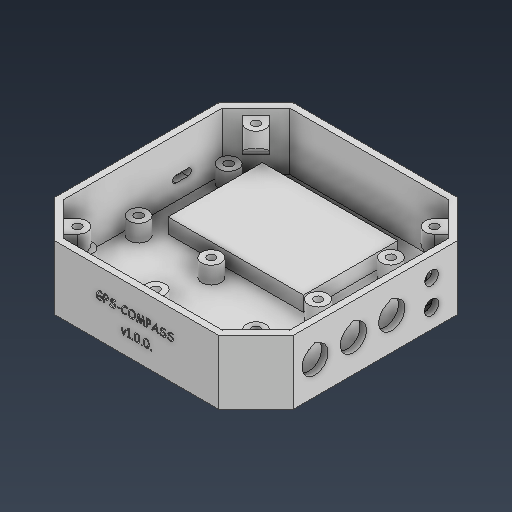
# Autodesk Inventor part: GPS-Compass_box
Saved by Autodesk Inventor 2026.2 (Build 302298000, 298)
## iProperties
Created: 2025-11-10
Part Number: GPS-Compass_box
Material: Generic
Document SubType Name: Modeling
Designer: MenMe
Density: 1 g/cm^3
Appearance: Default
Author: MenMe
Autodesk Inventor part; units mm, degrees
ref_plane "YZ Plane" through (0, 0, 0) normal (1, 0, 0) x (0, 1, 0)
ref_plane "XZ Plane" through (0, 0, 0) normal (0, 1, 0) x (-1, 0, 0)
ref_plane "XY Plane" through (0, 0, 0) normal (0, 0, 1) x (1, 0, 0)
sketch "Sketch1" plane through (0, 0, 0) normal (0, 1, 0) x (-1, 0, 0)
  line L0 (-56, 0) -> (56, 0) construction
  line L1 (0, 56) -> (0, -56) construction
  line L2 (56, 38.3223) -> (56, -38.3223)
  line L3 (56, 38.3223) -> (38.3223, 56)
  line L4 (38.3223, 56) -> (-38.3223, 56)
  line L5 (-38.3223, 56) -> (-56, 38.3223)
  line L6 (-56, 38.3223) -> (-56, -38.3223)
  line L7 (-56, -38.3223) -> (-38.3223, -56)
  line L8 (-38.3223, -56) -> (38.3223, -56)
  line L9 (38.3223, -56) -> (56, -38.3223)
  point P0 (0, 0)
  point P1 (0, 0)
  point P2 (56, 0)
  dimension "d0" = 112
  dimension "d1" = 112
  dimension "d2" = 135
  dimension "d3" = 135
  dimension "d4" = 135
  dimension "d8" = 25
  constraints: 20 end point, 7 midpoint, 2 horizontal, 2 perpendicular, 2 vertical, 1 coincident, 1 parallel
  measures "d0" distance of L0.start L0.end
  measures "d1" distance of L1.start L1.end
  measures "d2" angle of L2 L3
  measures "d3" angle of L2 L9
  measures "d4" angle of L5 L6
  measures "d8" distance of L6.end L7.end
extrude "Extrusion1" add sketch "Sketch1" along normal blind 30
sketch "Sketch2" plane through (0, 30, 0) normal (0, 1, 0) x (1, 0, 0)
  line L0 (38.3223, -56) -> (56, -38.3223) projected
  line L1 (56, -38.3223) -> (56, 38.3223) projected
  line L2 (56, 38.3223) -> (38.3223, 56) projected
  line L3 (38.3223, 56) -> (-38.3223, 56) projected
  line L4 (-38.3223, 56) -> (-56, 38.3223) projected
  line L5 (-56, 38.3223) -> (-56, -38.3223) projected
  line L6 (-56, -38.3223) -> (-38.3223, -56) projected
  line L7 (-38.3223, -56) -> (38.3223, -56) projected
  line L8 (-37.0797, 53) -> (37.0797, 53)
  line L9 (37.0797, 53) -> (53, 37.0797)
  line L10 (53, 37.0797) -> (53, -37.0797)
  line L11 (53, -37.0797) -> (37.0797, -53)
  line L12 (37.0797, -53) -> (-37.0797, -53)
  line L13 (-37.0797, -53) -> (-53, -37.0797)
  line L14 (-53, -37.0797) -> (-53, 37.0797)
  line L15 (-53, 37.0797) -> (-37.0797, 53)
  point P0 (0, 0)
  dimension "d11" = 3
  constraints: 16 end point, 7 other
  measures "d11" distance between parallel lines of L3 L8
extrude "Extrusion2" cut sketch "Sketch2" against normal blind 27 contours L8 L9 L10 L11 L12 L13 L14 L15
sketch "Sketch3" plane through (0, 3, 0) normal (0, 1, 0) x (1, 0, 0)
  circle A0 centre (-47.9582, 35.11) radius 4.5
  circle A1 centre (-47.9582, -7.09) radius 4.5
  circle A2 centre (-13.8582, -7.09) radius 4.5
  circle A3 centre (28.1418, 35.11) radius 4.5
  circle A4 centre (28.1418, 1.01) radius 4.5
  circle A5 centre (-14.0082, -33.0896) radius 4.5
  circle A6 centre (-47.8082, -33.0896) radius 4.5
  line L0 (-47.9582, -7.09) -> (-13.8582, -7.09) construction
  line L1 (-47.8082, -33.0896) -> (-14.0082, -33.0896) construction
  circle A7 centre (43.8518, 33.5) radius 4.5
  circle A8 centre (43.8518, -33.5) radius 4.5
  line L2 (37.0797, -53) -> (-37.0797, -53) projected
  line L3 (-53, -37.0797) -> (-53, 37.0797) projected
  line L4 (37.0797, 53) -> (53, 37.0797) projected
  line L5 (53, -37.0797) -> (37.0797, -53) projected
  line L6 (-10.6645, -2.1722) -> (28.1355, -2.1722)
  arc A9 (28.1355, -2.1722) -> (31.3355, 1.0278) centre (28.1355, 1.0278) ccw
  line L7 (31.3355, 35.1278) -> (31.3355, 1.0278)
  arc A10 (31.3355, 35.1278) -> (28.1355, 38.3278) centre (28.1355, 35.1278) ccw
  line L8 (6.8355, 38.3278) -> (28.1355, 38.3278)
  line L9 (6.8355, 32.6278) -> (6.8355, 38.3278)
  arc A11 (6.3355, 32.1278) -> (6.8355, 32.6278) centre (6.3355, 32.6278) ccw
  line L10 (-11.1645, 32.1278) -> (6.3355, 32.1278)
  arc A12 (-11.6645, 32.6278) -> (-11.1645, 32.1278) centre (-11.1645, 32.6278) ccw
  line L11 (-11.6645, 38.3278) -> (-11.6645, 32.6278)
  line L12 (-47.9645, 38.3278) -> (-11.6645, 38.3278)
  arc A13 (-47.9645, 38.3278) -> (-51.1645, 35.1278) centre (-47.9645, 35.1278) ccw
  line L13 (-51.1645, 35.1278) -> (-51.1645, 26.5778)
  arc A14 (-52.1645, 25.5778) -> (-51.1645, 26.5778) centre (-52.1645, 26.5778) ccw
  line L14 (-52.1645, 25.5778) -> (-52.6645, 25.5778)
  arc A15 (-52.6645, 25.5778) -> (-53.6645, 24.5778) centre (-52.6645, 24.5778) ccw
  line L15 (-53.6645, 24.5778) -> (-53.6645, 11.5778)
  arc A16 (-53.6645, 11.5778) -> (-52.6645, 10.5778) centre (-52.6645, 11.5778) ccw
  line L16 (-52.6645, 10.5778) -> (-52.1645, 10.5778)
  arc A17 (-51.1645, 9.5778) -> (-52.1645, 10.5778) centre (-52.1645, 9.5778) ccw
  line L17 (-51.1645, 9.5778) -> (-51.1645, -10.2722)
  line L18 (-51.1645, -10.2722) -> (-47.9645, -10.2722)
  arc A18 (-47.9645, -10.2722) -> (-44.7645, -7.0722) centre (-47.9645, -7.0722) ccw
  line L19 (-44.7645, -7.0722) -> (-44.7645, -6.6722)
  line L20 (-44.7645, -6.6722) -> (-17.0645, -6.6722)
  line L21 (-17.0645, -7.0722) -> (-17.0645, -6.6722)
  arc A19 (-17.0645, -7.0722) -> (-13.8645, -10.2722) centre (-13.8645, -7.0722) ccw
  line L22 (-13.8645, -10.2722) -> (-10.6645, -10.2722)
  line L23 (-10.6645, -2.1722) -> (-10.6645, -10.2722)
  line L24 (-51.1657, -10.3631) -> (-51.1657, -32.9831)
  arc A20 (-51.1657, -32.9831) -> (-47.8157, -36.3331) centre (-47.8157, -32.9831) ccw
  line L25 (-47.8157, -36.3331) -> (-14.0157, -36.3331)
  arc A21 (-14.0157, -36.3331) -> (-10.6657, -32.9831) centre (-14.0157, -32.9831) ccw
  line L26 (-10.6657, -10.3631) -> (-10.6657, -32.9831)
  line L27 (-10.6657, -10.3631) -> (-13.8657, -10.3631)
  arc A22 (-17.2157, -7.0131) -> (-13.8657, -10.3631) centre (-13.8657, -7.0131) ccw
  line L28 (-17.2157, -6.7631) -> (-17.2157, -7.0131)
  line L29 (-44.6157, -6.7631) -> (-17.2157, -6.7631)
  line L30 (-44.6157, -7.0131) -> (-44.6157, -6.7631)
  arc A23 (-47.9657, -10.3631) -> (-44.6157, -7.0131) centre (-47.9657, -7.0131) ccw
  line L31 (-51.1657, -10.3631) -> (-47.9657, -10.3631)
  arc A24 (38.8493, 37.5107) -> (36.8493, 35.5107) centre (38.8493, 35.5107) ccw
  line L32 (38.8493, 37.5107) -> (42.3493, 37.5107)
  line L33 (42.3493, 33.5107) -> (42.3493, 37.5107)
  arc A25 (42.3493, 33.5107) -> (45.3493, 33.5107) centre (43.8493, 33.5107) ccw
  line L34 (45.3493, 33.5107) -> (45.3493, 37.5107)
  line L35 (45.3493, 37.5107) -> (47.2531, 37.5107)
  line L36 (47.2531, 37.5107) -> (51.8493, 32.9145)
  line L37 (51.8493, -32.8931) -> (51.8493, 32.9145)
  line L38 (47.2531, -37.4893) -> (51.8493, -32.8931)
  line L39 (45.3493, -37.4893) -> (47.2531, -37.4893)
  line L40 (45.3493, -33.4893) -> (45.3493, -37.4893)
  arc A26 (45.3493, -33.4893) -> (42.3493, -33.4893) centre (43.8493, -33.4893) ccw
  line L41 (42.3493, -33.4893) -> (42.3493, -37.4893)
  line L42 (38.8493, -37.4893) -> (42.3493, -37.4893)
  arc A27 (36.8493, -35.4893) -> (38.8493, -37.4893) centre (38.8493, -35.4893) ccw
  line L43 (36.8493, 35.5107) -> (36.8493, -35.4893)
  point P0 (0, 0)
  point P1 (-30.9082, -33.0896)
  point P2 (-30.9082, -7.09)
  dimension "d40" = 9
  dimension "d43" = 34.1
  dimension "d58" = 76.1
  dimension "d59" = 42.2
  dimension "d60" = 34.1
  dimension "d90" = 33.8
  dimension "d105" = 26
  dimension "d128" = 9
  dimension "d135" = 67
  dimension "d144" = 34.51
  dimension "d147" = 15.71
  dimension "d264" = 9
  dimension "d265" = 9
  constraints: 80 end point, 38 point on circle, 28 centre point, 7 equal radius, 4 vertical alignment, 3 horizontal alignment, 2 horizontal, 2 midpoint
  measures "d40" diameter of A3
  measures "d43" distance of A3.centre A4.centre
  measures "d58" distance of A0.centre A3.centre
  measures "d59" distance of L0.start A0.centre
  measures "d60" distance of L0.end L0.start
  measures "d90" distance of L1.start L1.end
  measures "d105" distance of L1.end L0.end
  measures "d128" diameter of A5
  measures "d135" distance of A8.centre A7.centre
  measures "d144" vertical distance of A8.centre A4.centre
  measures "d147" horizontal distance of A7.centre A3.centre
  measures "d264" distance from line of L4 A7.centre
  measures "d265" distance from line of L5 A8.centre
extrude "Extrusion3" add sketch "Sketch3" along normal blind 8 contours A0 L13 A13 L12 | L12 A13 L13 A0 | L8 A10 L7 A3 | A3 L7 A10 L8 | L7 A9 L6 A4 | A4 L6 A9 L7 | L17 A1 | A1 L20 L19 A18 L18 L17 | A1 L29 L30 A23 L31 L18 A18 L19 L20 | A1 L31 A23 L30 L29 | L20 L21 A19 L22 A2 L27 A22 L28 L29 | A2 L23 L22 A19 L21 L20 | A2 L23 | L29 L28 A22 L27 A2 | L24 A20 L25 A6 | A6 L25 A20 L24 | L26 A21 L25 A5 | A5 L25 A21 L26 | A7 L32 L33 A25 L34 L35 | L35 L34 A25 L33 L32 A7 | L39 L40 A26 L41 L42 A8 | A8 L42 L41 A26 L40 L39
sketch "Sketch4" plane through (0, 3, 0) normal (0, 1, 0) x (1, 0, 0)
  line L0 (-41.4841, 44.4591) -> (22.0159, 44.4591)
  line L1 (22.0159, 44.4591) -> (22.0159, 0.2591)
  line L2 (22.0159, 0.2591) -> (-41.4841, 0.2591)
  line L3 (-41.4841, 0.2591) -> (-41.4841, 44.4591)
  point P0 (0, 0)
  dimension "d268" = 63.5
  dimension "d269" = 44.2
  constraints: 8 end point, 2 parallel, 1 horizontal, 1 perpendicular
  measures "d268" distance of L1.end L2.end
  measures "d269" distance of L0.end L1.end
extrude "Extrusion4" add sketch "Sketch4" along normal blind 7
sketch "Sketch5" plane through (-13.8582, 11, 7.09) normal (0, 1, 0) x (1, 0, 0)
  circle A0 centre (0, 0) radius 4.5 projected
  circle A1 centre (0, 0) radius 1.925
  circle A2 centre (-34.1, 0) radius 4.5 projected
  circle A3 centre (-34.1, 0) radius 1.925
  circle A4 centre (-34.1, 42.2) radius 4.5 projected
  circle A5 centre (-34.1, 42.2) radius 1.925
  circle A6 centre (42, 8.1) radius 4.5 projected
  circle A7 centre (42, 8.1) radius 1.925
  circle A8 centre (-33.95, -25.9996) radius 4.5 projected
  circle A9 centre (-33.95, -25.9996) radius 1.925
  circle A10 centre (-0.15, -25.9996) radius 4.5 projected
  circle A11 centre (-0.15, -25.9996) radius 1.925
  circle A12 centre (57.71, -26.41) radius 4.5 projected
  circle A13 centre (57.71, -26.41) radius 1.925
  circle A14 centre (57.71, 40.59) radius 4.5 projected
  circle A15 centre (57.71, 40.59) radius 1.925
  circle A16 centre (42, 42.2) radius 4.5 projected
  circle A17 centre (42, 42.2) radius 1.925
  point P0 (13.8582, 7.09)
  dimension "d272" = 3.85
  dimension "d273" = 3.85
  constraints: 9 centre point, 9 coincident, 7 equal radius
  measures "d272" diameter of A7
  measures "d273" diameter of A15
extrude "Extrusion5" cut sketch "Sketch5" against normal blind 5.3 contours A1 | A3 | A5 | A7 | A9 | A11 | A13 | A15 | A17
sketch "Sketch6" plane through (56, 0, 38.3223) normal (1, 0, 0) x (0, 0, -1)
  line L0 (76.6447, 0) -> (76.6447, 30) construction
  line L1 (76.6447, 15) -> (0, 15) construction
  line L2 (0, 0) -> (0, 30) construction
  arc A0 (7.0627, 20.4032) -> (12.9373, 20.4032) centre (10, 15) ccw
  line L3 (7.0627, 20.4032) -> (10, 22)
  line L4 (10, 22) -> (12.9373, 20.4032)
  arc A1 (25.0627, 20.4032) -> (30.9373, 20.4032) centre (28, 15) ccw
  line L5 (28, 22) -> (30.9373, 20.4032)
  line L6 (25.0627, 20.4032) -> (28, 22)
  arc A2 (43.0627, 20.4032) -> (48.9373, 20.4032) centre (46, 15) ccw
  line L7 (46, 22) -> (48.9373, 20.4032)
  line L8 (43.0627, 20.4032) -> (46, 22)
  circle A3 centre (64.6447, 21) radius 3.2
  circle A4 centre (64.6447, 9) radius 3.375
  point P0 (38.3223, 0)
  point P1 (52.15, 15)
  dimension "d276" = 12.3
  dimension "d277" = 7
  dimension "d280" = 18
  dimension "d285" = 10
  dimension "d288" = 6.75
  dimension "d289" = 6.4
  dimension "d290" = 12
  dimension "d291" = 6
  dimension "d292" = 6
  constraints: 14 end point, 7 point on circle, 5 centre point, 2 midpoint, 2 point on line, 2 tangent, 2 vertical alignment, 1 horizontal, 14 other
  measures "d276" diameter of A0
  measures "d277" distance of A0.centre L3.end
  measures "d280" distance of A0.centre A1.centre
  measures "d285" distance from line of L2 A0.centre
  measures "d288" diameter of A4
  measures "d289" diameter of A3
  measures "d290" distance from line of L0 A3.centre
  measures "d291" distance from line of L1 A3.centre
  measures "d292" distance from line of L1 A4.centre
extrude "Extrusion6" cut sketch "Sketch6" against normal blind 3
sketch "Sketch7" plane through (-56, 0, -38.3223) normal (-1, 0, 0) x (0, 0, 1)
  line L0 (0, 0) -> (0, 30) construction
  line L1 (76.6447, 0) -> (76.6447, 30) construction
  line L2 (17.16, 12) -> (22.84, 12) construction
  line L3 (17.16, 10.37) -> (22.84, 10.37)
  line L4 (22.84, 13.63) -> (17.16, 13.63)
  arc A0 (17.16, 13.63) -> (17.16, 10.37) centre (17.16, 12) ccw
  arc A1 (22.84, 10.37) -> (22.84, 13.63) centre (22.84, 12) ccw
  line L5 (0, 0) -> (76.6447, 0) projected
  point P0 (38.3223, 0)
  point P1 (20, 12)
  dimension "d297" = 8.94
  dimension "d298" = 3.26
  dimension "d299" = 12
  dimension "d302" = 20
  constraints: 8 end point, 4 point on circle, 4 tangent, 2 centre point, 1 horizontal, 1 midpoint, 1 parallel
  measures "d298" distance between parallel lines of L3 L4
  measures "d299" distance from line of L5 point (20, 12)
  measures "d302" distance from line of L0 point (20, 12)
extrude "Extrusion7" cut sketch "Sketch7" against normal blind 3
ref_plane "Work Plane2" through (0, 27, 0) normal (0, 1, 0) x (1, 0, 0)
sketch "Sketch8" plane through (0, 27, 0) normal (0, 1, 0) x (1, 0, 0)
  line L0 (-53, 37.0797) -> (-37.0797, 53) construction
  line L1 (-45.0398, 45.0398) -> (45.0398, -45.0398) construction
  line L2 (53, -37.0797) -> (37.0797, -53) projected
  line L3 (37.0797, 53) -> (53, 37.0797) construction
  line L4 (45.0398, 45.0398) -> (-45.0398, -45.0398) construction
  arc A0 (-45.0398, 38.6759) -> (-38.6759, 45.0398) centre (-41.8579, 41.8579) ccw
  arc A1 (38.6759, 45.0398) -> (45.0398, 38.6759) centre (41.8579, 41.8579) ccw
  arc A2 (-38.6759, -45.0398) -> (-45.0398, -38.6759) centre (-41.8579, -41.8579) ccw
  arc A3 (45.0398, -38.6759) -> (38.6759, -45.0398) centre (41.8579, -41.8579) ccw
  line L5 (-37.0797, -53) -> (-53, -37.0797) projected
  line L6 (-45.0398, 38.6759) -> (-48.2218, 41.8579)
  line L7 (-38.6759, 45.0398) -> (-41.8579, 48.2218)
  line L8 (45.0398, 38.6759) -> (48.2218, 41.8579)
  line L9 (38.6759, 45.0398) -> (41.8579, 48.2218)
  line L10 (38.6759, -45.0398) -> (41.8579, -48.2218)
  line L11 (45.0398, -38.6759) -> (48.2218, -41.8579)
  line L12 (-45.0398, -38.6759) -> (-48.2218, -41.8579)
  line L13 (-38.6759, -45.0398) -> (-41.8579, -48.2218)
  line L14 (-53, 37.0797) -> (-37.0797, 53) projected
  line L15 (37.0797, 53) -> (53, 37.0797) projected
  point P0 (0, 0)
  dimension "d303" = 9
  constraints: 20 end point, 14 point on line, 11 tangent, 8 perpendicular, 8 point on circle, 6 midpoint, 4 centre point, 3 equal radius
  measures "d303" diameter of A0
extrude "Extrusion8" add sketch "Sketch8" against normal blind 7
chamfer "Chamfer1" distance 8.99 angle 45 4 edges at (45.0398, 20, -45.0398) (45.0398, 20, 45.0398) (-45.0398, 20, 45.0398) (-45.0398, 20, -45.0398)
sketch "Sketch9" plane through (0, 27, 0) normal (0, 1, 0) x (1, 0, 0)
  arc A0 (-38.895, 38.4709) -> (-38.4709, 38.895) centre (-41.8579, 41.8579) ccw projected
  circle A1 centre (-41.8579, 41.8579) radius 1.925
  arc A2 (38.4709, 38.895) -> (38.895, 38.4709) centre (41.8579, 41.8579) ccw projected
  circle A3 centre (41.8579, 41.8579) radius 1.925
  arc A4 (-38.6759, -45.0398) -> (-45.0398, -38.6759) centre (-41.8579, -41.8579) ccw projected
  circle A5 centre (-41.8579, -41.8579) radius 1.925
  arc A6 (38.895, -38.4709) -> (38.4709, -38.895) centre (41.8579, -41.8579) ccw projected
  circle A7 centre (41.8579, -41.8579) radius 1.925
  point P0 (0, 0)
  dimension "d310" = 3.85
  constraints: 4 centre point, 4 coincident, 3 equal radius
  measures "d310" diameter of A5
extrude "Extrusion9" cut sketch "Sketch9" against normal blind 5.4
sketch "Sketch10" plane through (-38.3223, 0, 56) normal (0, 0, 1) x (1, 0, 0)
  line L0 (18.3223, 22) -> (58.3223, 22) construction
  line L1 (58.3223, 22) -> (58.3223, 6) construction
  line L2 (58.3223, 6) -> (18.3223, 6) construction
  line L3 (18.3223, 6) -> (18.3223, 22) construction
  line L4 (0, 30) -> (76.6447, 30) construction
  line L5 (38.3223, 30) -> (38.3223, 0) construction
  line L6 (76.6447, 0) -> (76.6447, 30) construction
  line L7 (76.6447, 15) -> (0, 15) construction
  line L8 (0, 0) -> (0, 30) construction
  line L9 (0, 0) -> (76.6447, 0) construction
  spline S0 degree 2 poles (22.462, 17.9114) (22.3103, 17.1528) (21.3275, 16.2459) (20.6585, 16.2459) knots 0 0 0 1 2 2 2
  spline S1 degree 2 poles (20.6585, 16.2459) (20.0482, 16.2459) (19.4413, 16.9252) (19.4413, 17.608) knots 0 0 0 1 2 2 2
  spline S2 degree 2 poles (19.4413, 17.608) (19.4413, 18.2494) (20.0482, 19.608) (20.5241, 20.0252) knots 0 0 0 1 2 2 2
  spline S3 degree 2 poles (20.5241, 20.0252) (20.8413, 20.3045) (21.193, 20.3045) knots 0 0 0 1 1 1
  spline S4 degree 2 poles (21.193, 20.3045) (21.4172, 20.3045) (21.7861, 20.1563) knots 0 0 0 1 1 1
  spline S5 degree 2 poles (21.7861, 20.1563) (22.2378, 19.977) (22.2378, 19.7632) knots 0 0 0 1 1 1
  spline S6 degree 2 poles (22.2378, 19.7632) (22.2378, 19.6597) (22.0896, 19.5011) (21.9861, 19.5011) knots 0 0 0 1 2 2 2
  spline S7 degree 2 poles (21.9861, 19.5011) (21.931, 19.5011) (21.831, 19.5632) knots 0 0 0 1 1 1
  spline S8 degree 2 poles (21.831, 19.5632) (21.4551, 19.7942) (21.193, 19.7942) knots 0 0 0 1 1 1
  spline S9 degree 2 poles (21.193, 19.7942) (21.0068, 19.7942) (20.8034, 19.6011) knots 0 0 0 1 1 1
  spline S10 degree 2 poles (20.8034, 19.6011) (20.7034, 19.5045) (20.5137, 19.2494) knots 0 0 0 1 1 1
  spline S11 degree 2 poles (20.5137, 19.2494) (19.9413, 18.4942) (19.9413, 17.608) knots 0 0 0 1 1 1
  spline S12 degree 2 poles (19.9413, 17.608) (19.9413, 17.1425) (20.0861, 16.9563) knots 0 0 0 1 1 1
  spline S13 degree 2 poles (20.0861, 16.9563) (20.2413, 16.7528) (20.6585, 16.7528) knots 0 0 0 1 1 1
  spline S14 degree 2 poles (20.6585, 16.7528) (21.0999, 16.7528) (21.4275, 17.0321) knots 0 0 0 1 1 1
  spline S15 degree 2 poles (21.4275, 17.0321) (21.7723, 17.3287) (21.9068, 17.8804) knots 0 0 0 1 1 1
  spline S16 degree 2 poles (21.9068, 17.8804) (21.2241, 17.8459) (20.7344, 17.6183) knots 0 0 0 1 1 1
  spline S17 degree 2 poles (20.7344, 17.6183) (20.6758, 17.5907) (20.6241, 17.5907) knots 0 0 0 1 1 1
  spline S18 degree 2 poles (20.6241, 17.5907) (20.5137, 17.5907) (20.4413, 17.6735) knots 0 0 0 1 1 1
  spline S19 degree 2 poles (20.4413, 17.6735) (20.3758, 17.7528) (20.3758, 17.8528) knots 0 0 0 1 1 1
  spline S20 degree 2 poles (20.3758, 17.8528) (20.3758, 17.9873) (20.5068, 18.0701) knots 0 0 0 1 1 1
  spline S21 degree 2 poles (20.5068, 18.0701) (21.0413, 18.3942) (22.3482, 18.3942) knots 0 0 0 1 1 1
  spline S22 degree 2 poles (22.3482, 18.3942) (22.4516, 18.3942) (22.5965, 18.2494) (22.5965, 18.1425) knots 0 0 0 1 2 2 2
  spline S23 degree 2 poles (22.5965, 18.1425) (22.5965, 17.9804) (22.462, 17.9114) knots 0 0 0 1 1 1
  spline S24 degree 2 poles (23.7068, 17.8701) (23.6378, 17.8701) (23.4034, 17.9011) knots 0 0 0 1 1 1
  spline S25 degree 2 poles (23.4034, 17.9011) (23.3861, 17.5287) (23.3861, 16.5942) knots 0 0 0 1 1 1
  spline S26 degree 2 poles (23.3861, 16.5942) (23.3861, 16.4942) (23.2585, 16.3597) (23.162, 16.3597) knots 0 0 0 1 2 2 2
  spline S27 degree 2 poles (23.162, 16.3597) (23.062, 16.3597) (22.9344, 16.4942) (22.9344, 16.5942) knots 0 0 0 1 2 2 2
  line L10 (22.9344, 16.5942) -> (22.9344, 17.3218)
  spline S28 degree 2 poles (22.9344, 17.3218) (22.9344, 17.6838) (22.9792, 18.3459) knots 0 0 0 1 1 1
  spline S29 degree 2 poles (22.9792, 18.3459) (23.0275, 19.0597) (23.031, 19.3701) knots 0 0 0 1 1 1
  line L11 (23.031, 19.3701) -> (23.031, 19.7114)
  spline S30 degree 2 poles (23.031, 19.7114) (23.031, 19.9563) (23.062, 20.0666) knots 0 0 0 1 1 1
  spline S31 degree 2 poles (23.062, 20.0666) (23.1206, 20.2838) (23.3034, 20.2563) knots 0 0 0 1 1 1
  spline S32 degree 2 poles (23.3034, 20.2563) (23.3827, 20.2804) (23.6758, 20.3045) (23.8896, 20.3045) knots 0 0 0 1 2 2 2
  spline S33 degree 2 poles (23.8896, 20.3045) (24.3413, 20.3045) (24.7378, 19.9942) knots 0 0 0 1 1 1
  spline S34 degree 2 poles (24.7378, 19.9942) (25.1723, 19.6528) (25.1723, 19.1735) knots 0 0 0 1 1 1
  spline S35 degree 2 poles (25.1723, 19.1735) (25.1723, 18.5597) (24.7068, 18.1976) knots 0 0 0 1 1 1
  spline S36 degree 2 poles (24.7068, 18.1976) (24.2896, 17.8701) (23.7068, 17.8701) knots 0 0 0 1 1 1
  spline S37 degree 2 poles (23.831, 19.8356) (23.7206, 19.8356) (23.5482, 19.8252) (23.4896, 19.8149) knots 0 0 0 1 2 2 2
  line L12 (23.4896, 19.8149) -> (23.4861, 19.3597)
  line L13 (23.4861, 19.3597) -> (23.4344, 18.3735)
  line L14 (23.4344, 18.3735) -> (23.7068, 18.3425)
  spline S38 degree 2 poles (23.7068, 18.3425) (24.1241, 18.3425) (24.4068, 18.5528) knots 0 0 0 1 1 1
  spline S39 degree 2 poles (24.4068, 18.5528) (24.7206, 18.7838) (24.7206, 19.1735) knots 0 0 0 1 1 1
  spline S40 degree 2 poles (24.7206, 19.1735) (24.7206, 19.4528) (24.4241, 19.6528) knots 0 0 0 1 1 1
  spline S41 degree 2 poles (24.4241, 19.6528) (24.1482, 19.8356) (23.831, 19.8356) knots 0 0 0 1 1 1
  spline S42 degree 2 poles (25.6585, 17.0321) (25.6551, 17.1356) (25.8034, 17.2666) (25.9068, 17.2666) knots 0 0 0 1 2 2 2
  spline S43 degree 2 poles (25.9068, 17.2666) (26.0275, 17.2666) (26.1206, 17.1287) knots 0 0 0 1 1 1
  spline S44 degree 2 poles (26.1206, 17.1287) (26.2482, 16.939) (26.3447, 16.8735) knots 0 0 0 1 1 1
  spline S45 degree 2 poles (26.3447, 16.8735) (26.5551, 16.7356) (26.9551, 16.7356) knots 0 0 0 1 1 1
  spline S46 degree 2 poles (26.9551, 16.7356) (27.3413, 16.7356) (27.6689, 16.9011) knots 0 0 0 1 1 1
  spline S47 degree 2 poles (27.6689, 16.9011) (28.0896, 17.1149) (28.0896, 17.4907) knots 0 0 0 1 1 1
  spline S48 degree 2 poles (28.0896, 17.4907) (28.0896, 17.8045) (27.7344, 17.9838) knots 0 0 0 1 1 1
  spline S49 degree 2 poles (27.7344, 17.9838) (27.4378, 18.139) (26.9965, 18.1528) knots 0 0 0 1 1 1
  spline S50 degree 2 poles (26.9965, 18.1528) (26.6068, 18.1666) (26.331, 18.3252) knots 0 0 0 1 1 1
  spline S51 degree 2 poles (26.331, 18.3252) (25.9792, 18.5252) (25.9792, 18.8976) knots 0 0 0 1 1 1
  spline S52 degree 2 poles (25.9792, 18.8976) (25.9792, 19.339) (26.4792, 19.7011) knots 0 0 0 1 1 1
  spline S53 degree 2 poles (26.4792, 19.7011) (26.9551, 20.0459) (27.4654, 20.0459) knots 0 0 0 1 1 1
  spline S54 degree 2 poles (27.4654, 20.0459) (27.7034, 20.0459) (28.0068, 19.9632) knots 0 0 0 1 1 1
  spline S55 degree 2 poles (28.0068, 19.9632) (28.4068, 19.8563) (28.4068, 19.6907) knots 0 0 0 1 1 1
  spline S56 degree 2 poles (28.4068, 19.6907) (28.4068, 19.4735) (28.1861, 19.4735) knots 0 0 0 1 1 1
  spline S57 degree 2 poles (28.1861, 19.4735) (28.0861, 19.4735) (27.593, 19.5804) (27.4551, 19.577) knots 0 0 0 1 2 2 2
  spline S58 degree 2 poles (27.4551, 19.577) (27.0689, 19.5735) (26.7999, 19.3873) knots 0 0 0 1 1 1
  spline S59 degree 2 poles (26.7999, 19.3873) (26.5241, 19.1976) (26.5241, 18.9252) knots 0 0 0 1 1 1
  spline S60 degree 2 poles (26.5241, 18.9252) (26.5241, 18.7218) (26.8896, 18.6356) knots 0 0 0 1 1 1
  spline S61 degree 2 poles (26.8896, 18.6356) (27.0275, 18.6045) (27.4172, 18.577) knots 0 0 0 1 1 1
  spline S62 degree 2 poles (27.4172, 18.577) (27.9827, 18.5356) (28.2999, 18.2218) knots 0 0 0 1 1 1
  spline S63 degree 2 poles (28.2999, 18.2218) (28.593, 17.9356) (28.593, 17.5218) knots 0 0 0 1 1 1
  spline S64 degree 2 poles (28.593, 17.5218) (28.593, 16.9321) (28.0482, 16.5804) knots 0 0 0 1 1 1
  spline S65 degree 2 poles (28.0482, 16.5804) (27.5758, 16.277) (26.9551, 16.277) knots 0 0 0 1 1 1
  spline S66 degree 2 poles (26.9551, 16.277) (26.4999, 16.277) (26.1275, 16.4494) knots 0 0 0 1 1 1
  spline S67 degree 2 poles (26.1275, 16.4494) (25.6654, 16.6632) (25.6585, 17.0321) knots 0 0 0 1 1 1
  spline S68 degree 2 poles (30.5172, 17.5942) (30.1827, 17.5597) (29.3206, 17.5597) knots 0 0 0 1 1 1
  spline S69 degree 2 poles (29.3206, 17.5597) (29.1137, 17.5597) (29.1137, 17.7528) knots 0 0 0 1 1 1
  spline S70 degree 2 poles (29.1137, 17.7528) (29.1137, 17.9459) (29.3206, 17.9459) knots 0 0 0 1 1 1
  spline S71 degree 2 poles (29.3206, 17.9459) (29.5172, 17.9459) (30.2999, 17.9804) (30.493, 17.9804) knots 0 0 0 1 2 2 2
  spline S72 degree 2 poles (30.493, 17.9804) (30.7137, 17.9804) (30.7137, 17.7873) knots 0 0 0 1 1 1
  spline S73 degree 2 poles (30.7137, 17.7873) (30.7137, 17.6183) (30.5172, 17.5942) knots 0 0 0 1 1 1
  spline S74 degree 2 poles (33.6792, 19.1907) (33.5206, 19.1907) (33.4413, 19.377) knots 0 0 0 1 1 1
  spline S75 degree 2 poles (33.4413, 19.377) (33.3723, 19.5356) (33.3137, 19.5701) knots 0 0 0 1 1 1
  spline S76 degree 2 poles (33.3137, 19.5701) (33.262, 19.5976) (33.0551, 19.5976) knots 0 0 0 1 1 1
  spline S77 degree 2 poles (33.0551, 19.5976) (32.6965, 19.5976) (32.2585, 19.0494) knots 0 0 0 1 1 1
  spline S78 degree 2 poles (32.2585, 19.0494) (31.6654, 18.3114) (31.6654, 17.6528) knots 0 0 0 1 1 1
  spline S79 degree 2 poles (31.6654, 17.6528) (31.6654, 17.3321) (31.8723, 17.1045) knots 0 0 0 1 1 1
  spline S80 degree 2 poles (31.8723, 17.1045) (32.0827, 16.8666) (32.3792, 16.8666) knots 0 0 0 1 1 1
  spline S81 degree 2 poles (32.3792, 16.8666) (32.6344, 16.8666) (32.8896, 16.9976) knots 0 0 0 1 1 1
  spline S82 degree 2 poles (32.8896, 16.9976) (33.0344, 17.0735) (33.331, 17.2907) knots 0 0 0 1 1 1
  spline S83 degree 2 poles (33.331, 17.2907) (33.4723, 17.3942) (33.5447, 17.3942) knots 0 0 0 1 1 1
  spline S84 degree 2 poles (33.5447, 17.3942) (33.6482, 17.3942) (33.793, 17.2321) (33.793, 17.1356) knots 0 0 0 1 2 2 2
  spline S85 degree 2 poles (33.793, 17.1356) (33.793, 17.0218) (33.6999, 16.939) knots 0 0 0 1 1 1
  spline S86 degree 2 poles (33.6999, 16.939) (33.0447, 16.3597) (32.3792, 16.3597) knots 0 0 0 1 1 1
  spline S87 degree 2 poles (32.3792, 16.3597) (31.8654, 16.3597) (31.5137, 16.7528) knots 0 0 0 1 1 1
  spline S88 degree 2 poles (31.5137, 16.7528) (31.1723, 17.1321) (31.1723, 17.6528) knots 0 0 0 1 1 1
  spline S89 degree 2 poles (31.1723, 17.6528) (31.1723, 18.4907) (31.8758, 19.3701) knots 0 0 0 1 1 1
  spline S90 degree 2 poles (31.8758, 19.3701) (32.462, 20.1045) (33.0551, 20.1045) knots 0 0 0 1 1 1
  spline S91 degree 2 poles (33.0551, 20.1045) (33.1758, 20.1045) (33.3689, 20.0838) (33.4447, 20.0563) knots 0 0 0 1 2 2 2
  spline S92 degree 2 poles (33.4447, 20.0563) (33.531, 20.1838) (33.6689, 20.1838) knots 0 0 0 1 1 1
  spline S93 degree 2 poles (33.6689, 20.1838) (33.8413, 20.1838) (33.8861, 19.9597) knots 0 0 0 1 1 1
  spline S94 degree 2 poles (33.8861, 19.9597) (33.9241, 19.7563) (33.9241, 19.4666) knots 0 0 0 1 1 1
  spline S95 degree 2 poles (33.9241, 19.4666) (33.9241, 19.3632) (33.8689, 19.2873) knots 0 0 0 1 1 1
  spline S96 degree 2 poles (33.8689, 19.2873) (33.8034, 19.1907) (33.6792, 19.1907) knots 0 0 0 1 1 1
  spline S97 degree 2 poles (35.9827, 16.2666) (35.2861, 16.2666) (34.7999, 16.6838) knots 0 0 0 1 1 1
  spline S98 degree 2 poles (34.7999, 16.6838) (34.2861, 17.1287) (34.2861, 17.8321) knots 0 0 0 1 1 1
  spline S99 degree 2 poles (34.2861, 17.8321) (34.2861, 18.6907) (34.793, 19.3907) knots 0 0 0 1 1 1
  spline S100 degree 2 poles (34.793, 19.3907) (35.3585, 20.1666) (36.2068, 20.1666) knots 0 0 0 1 1 1
  spline S101 degree 2 poles (36.2068, 20.1666) (37.0172, 20.1666) (37.4137, 19.8011) knots 0 0 0 1 1 1
  spline S102 degree 2 poles (37.4137, 19.8011) (37.8275, 19.4183) (37.8275, 18.5976) knots 0 0 0 1 1 1
  spline S103 degree 2 poles (37.8275, 18.5976) (37.8275, 17.7425) (37.362, 17.0528) knots 0 0 0 1 1 1
  spline S104 degree 2 poles (37.362, 17.0528) (36.8275, 16.2666) (35.9827, 16.2666) knots 0 0 0 1 1 1
  spline S105 degree 2 poles (36.2068, 19.6597) (35.5999, 19.6597) (35.1792, 19.0563) knots 0 0 0 1 1 1
  spline S106 degree 2 poles (35.1792, 19.0563) (34.7896, 18.5011) (34.7896, 17.8321) knots 0 0 0 1 1 1
  spline S107 degree 2 poles (34.7896, 17.8321) (34.7896, 17.3563) (35.1447, 17.0563) knots 0 0 0 1 1 1
  spline S108 degree 2 poles (35.1447, 17.0563) (35.4827, 16.7735) (35.9827, 16.7735) knots 0 0 0 1 1 1
  spline S109 degree 2 poles (35.9827, 16.7735) (36.5827, 16.7735) (36.9758, 17.3804) knots 0 0 0 1 1 1
  spline S110 degree 2 poles (36.9758, 17.3804) (37.3241, 17.9218) (37.3241, 18.5976) knots 0 0 0 1 1 1
  spline S111 degree 2 poles (37.3241, 18.5976) (37.3241, 19.1907) (37.0585, 19.4287) knots 0 0 0 1 1 1
  spline S112 degree 2 poles (37.0585, 19.4287) (36.8068, 19.6597) (36.2068, 19.6597) knots 0 0 0 1 1 1
  spline S113 degree 2 poles (42.062, 16.2114) (41.9275, 16.2114) (41.8413, 16.3494) knots 0 0 0 1 1 1
  spline S114 degree 2 poles (41.8413, 16.3494) (41.7689, 16.4701) (41.7103, 16.7459) knots 0 0 0 1 1 1
  line L15 (41.7103, 16.7459) -> (41.6206, 17.1735)
  spline S115 degree 2 poles (41.6206, 17.1735) (41.5172, 17.5701) (41.2999, 18.9183) knots 0 0 0 1 1 1
  line L16 (41.2999, 18.9183) -> (40.8034, 17.4287)
  line L17 (40.8034, 17.4287) -> (40.6585, 16.9563)
  spline S116 degree 2 poles (40.6585, 16.9563) (40.5689, 16.677) (40.4723, 16.5011) knots 0 0 0 1 1 1
  spline S117 degree 2 poles (40.4723, 16.5011) (40.3689, 16.3114) (40.193, 16.3114) knots 0 0 0 1 1 1
  spline S118 degree 2 poles (40.193, 16.3114) (40.0447, 16.3114) (39.962, 16.4701) knots 0 0 0 1 1 1
  spline S119 degree 2 poles (39.962, 16.4701) (39.9068, 16.5735) (39.862, 16.7356) knots 0 0 0 1 1 1
  line L18 (39.862, 16.7356) -> (39.7896, 17.008)
  spline S120 degree 2 poles (39.7896, 17.008) (39.5413, 17.8838) (39.3516, 18.8804) knots 0 0 0 1 1 1
  line L19 (39.3516, 18.8804) -> (39.262, 18.4356)
  line L20 (39.262, 18.4356) -> (38.9413, 17.1287)
  spline S121 degree 2 poles (38.9413, 17.1287) (38.9241, 16.9011) (38.8206, 16.4494) knots 0 0 0 1 1 1
  spline S122 degree 2 poles (38.8206, 16.4494) (38.7447, 16.2563) (38.5758, 16.2563) knots 0 0 0 1 1 1
  spline S123 degree 2 poles (38.5758, 16.2563) (38.4551, 16.2563) (38.3827, 16.3425) knots 0 0 0 1 1 1
  spline S124 degree 2 poles (38.3827, 16.3425) (38.3206, 16.4183) (38.3206, 16.5252) knots 0 0 0 1 1 1
  spline S125 degree 2 poles (38.3206, 16.5252) (38.3206, 16.939) (38.4896, 17.5425) knots 0 0 0 1 1 1
  line L21 (38.4896, 17.5425) -> (38.762, 18.539)
  line L22 (38.762, 18.539) -> (38.9068, 19.3183)
  spline S126 degree 2 poles (38.9068, 19.3183) (39.0137, 19.8666) (39.1344, 20.0321) knots 0 0 0 1 1 1
  spline S127 degree 2 poles (39.1344, 20.0321) (39.2344, 20.177) (39.3792, 20.177) knots 0 0 0 1 1 1
  spline S128 degree 2 poles (39.3792, 20.177) (39.5413, 20.177) (39.6206, 19.9942) knots 0 0 0 1 1 1
  spline S129 degree 2 poles (39.6206, 19.9942) (39.7172, 19.7735) (39.8275, 19.0942) knots 0 0 0 1 1 1
  spline S130 degree 2 poles (39.8275, 19.0942) (39.9585, 18.2804) (40.2378, 17.3321) knots 0 0 0 1 1 1
  spline S131 degree 2 poles (40.2378, 17.3321) (40.6034, 18.2873) (40.8689, 19.3183) knots 0 0 0 1 1 1
  line L23 (40.8689, 19.3183) -> (40.9447, 19.6804)
  spline S132 degree 2 poles (40.9447, 19.6804) (40.9896, 19.8976) (41.062, 20.0321) knots 0 0 0 1 1 1
  spline S133 degree 2 poles (41.062, 20.0321) (41.1585, 20.2114) (41.3241, 20.2114) knots 0 0 0 1 1 1
  spline S134 degree 2 poles (41.3241, 20.2114) (41.5378, 20.2114) (41.6482, 19.8045) knots 0 0 0 1 1 1
  spline S135 degree 2 poles (41.6482, 19.8045) (41.6896, 19.6632) (41.7447, 19.2183) knots 0 0 0 1 1 1
  spline S136 degree 2 poles (41.7447, 19.2183) (41.893, 18.1011) (42.1103, 17.308) knots 0 0 0 1 1 1
  line L24 (42.1103, 17.308) -> (42.231, 16.8838)
  spline S137 degree 2 poles (42.231, 16.8838) (42.3241, 16.5425) (42.3241, 16.4632) knots 0 0 0 1 1 1
  spline S138 degree 2 poles (42.3241, 16.4632) (42.3241, 16.3563) (42.162, 16.2114) (42.062, 16.2114) knots 0 0 0 1 2 2 2
  spline S139 degree 2 poles (43.5378, 17.8701) (43.4689, 17.8701) (43.2344, 17.9011) knots 0 0 0 1 1 1
  spline S140 degree 2 poles (43.2344, 17.9011) (43.2172, 17.5287) (43.2172, 16.5942) knots 0 0 0 1 1 1
  spline S141 degree 2 poles (43.2172, 16.5942) (43.2172, 16.4942) (43.0896, 16.3597) (42.993, 16.3597) knots 0 0 0 1 2 2 2
  spline S142 degree 2 poles (42.993, 16.3597) (42.893, 16.3597) (42.7654, 16.4942) (42.7654, 16.5942) knots 0 0 0 1 2 2 2
  line L25 (42.7654, 16.5942) -> (42.7654, 17.3218)
  spline S143 degree 2 poles (42.7654, 17.3218) (42.7654, 17.6838) (42.8103, 18.3459) knots 0 0 0 1 1 1
  spline S144 degree 2 poles (42.8103, 18.3459) (42.8585, 19.0597) (42.862, 19.3701) knots 0 0 0 1 1 1
  line L26 (42.862, 19.3701) -> (42.862, 19.7114)
  spline S145 degree 2 poles (42.862, 19.7114) (42.862, 19.9563) (42.893, 20.0666) knots 0 0 0 1 1 1
  spline S146 degree 2 poles (42.893, 20.0666) (42.9516, 20.2838) (43.1344, 20.2563) knots 0 0 0 1 1 1
  spline S147 degree 2 poles (43.1344, 20.2563) (43.2137, 20.2804) (43.5068, 20.3045) (43.7206, 20.3045) knots 0 0 0 1 2 2 2
  spline S148 degree 2 poles (43.7206, 20.3045) (44.1723, 20.3045) (44.5689, 19.9942) knots 0 0 0 1 1 1
  spline S149 degree 2 poles (44.5689, 19.9942) (45.0034, 19.6528) (45.0034, 19.1735) knots 0 0 0 1 1 1
  spline S150 degree 2 poles (45.0034, 19.1735) (45.0034, 18.5597) (44.5378, 18.1976) knots 0 0 0 1 1 1
  spline S151 degree 2 poles (44.5378, 18.1976) (44.1206, 17.8701) (43.5378, 17.8701) knots 0 0 0 1 1 1
  spline S152 degree 2 poles (43.662, 19.8356) (43.5516, 19.8356) (43.3792, 19.8252) (43.3206, 19.8149) knots 0 0 0 1 2 2 2
  line L27 (43.3206, 19.8149) -> (43.3172, 19.3597)
  line L28 (43.3172, 19.3597) -> (43.2654, 18.3735)
  line L29 (43.2654, 18.3735) -> (43.5378, 18.3425)
  spline S153 degree 2 poles (43.5378, 18.3425) (43.9551, 18.3425) (44.2378, 18.5528) knots 0 0 0 1 1 1
  spline S154 degree 2 poles (44.2378, 18.5528) (44.5516, 18.7838) (44.5516, 19.1735) knots 0 0 0 1 1 1
  spline S155 degree 2 poles (44.5516, 19.1735) (44.5516, 19.4528) (44.2551, 19.6528) knots 0 0 0 1 1 1
  spline S156 degree 2 poles (44.2551, 19.6528) (43.9792, 19.8356) (43.662, 19.8356) knots 0 0 0 1 1 1
  spline S157 degree 2 poles (48.2482, 16.3425) (48.0206, 16.3425) (47.8516, 16.9252) knots 0 0 0 1 1 1
  spline S158 degree 2 poles (47.8516, 16.9252) (47.7861, 17.1494) (47.6896, 17.7045) knots 0 0 0 1 1 1
  spline S159 degree 2 poles (47.6896, 17.7045) (47.4378, 17.6701) (47.031, 17.5804) knots 0 0 0 1 1 1
  line L30 (47.031, 17.5804) -> (46.3758, 17.4459)
  spline S160 degree 2 poles (46.3758, 17.4459) (46.2516, 17.1218) (45.9482, 16.4976) knots 0 0 0 1 1 1
  spline S161 degree 2 poles (45.9482, 16.4976) (45.8689, 16.3597) (45.7344, 16.3597) knots 0 0 0 1 1 1
  spline S162 degree 2 poles (45.7344, 16.3597) (45.6344, 16.3597) (45.4792, 16.5045) (45.4792, 16.608) knots 0 0 0 1 2 2 2
  spline S163 degree 2 poles (45.4792, 16.608) (45.4792, 16.7287) (45.8516, 17.5114) knots 0 0 0 1 1 1
  spline S164 degree 2 poles (45.8516, 17.5114) (45.8103, 17.577) (45.8103, 17.6597) knots 0 0 0 1 1 1
  spline S165 degree 2 poles (45.8103, 17.6597) (45.8103, 17.8597) (46.0516, 17.9183) knots 0 0 0 1 1 1
  spline S166 degree 2 poles (46.0516, 17.9183) (46.3344, 18.4459) (46.7654, 19.1356) knots 0 0 0 1 1 1
  spline S167 degree 2 poles (46.7654, 19.1356) (47.3516, 20.0735) (47.4965, 20.0735) knots 0 0 0 1 1 1
  spline S168 degree 2 poles (47.4965, 20.0735) (47.6896, 20.0735) (47.762, 19.8011) knots 0 0 0 1 1 1
  line L31 (47.762, 19.8011) -> (47.9172, 18.9701)
  line L32 (47.9172, 18.9701) -> (48.2861, 17.2494)
  line L33 (48.2861, 17.2494) -> (48.4275, 16.8597)
  spline S169 degree 2 poles (48.4275, 16.8597) (48.4999, 16.6597) (48.4999, 16.5907) knots 0 0 0 1 1 1
  spline S170 degree 2 poles (48.4999, 16.5907) (48.4999, 16.4873) (48.3482, 16.3425) (48.2482, 16.3425) knots 0 0 0 1 2 2 2
  line L34 (47.3758, 19.1701) -> (46.6689, 18.0287)
  spline S171 degree 2 poles (46.6689, 18.0287) (46.9689, 18.1045) (47.5758, 18.2149) knots 0 0 0 1 1 1
  line L35 (47.5758, 18.2149) -> (47.3758, 19.1701)
  spline S172 degree 2 poles (49.193, 17.0321) (49.1896, 17.1356) (49.3378, 17.2666) (49.4413, 17.2666) knots 0 0 0 1 2 2 2
  spline S173 degree 2 poles (49.4413, 17.2666) (49.562, 17.2666) (49.6551, 17.1287) knots 0 0 0 1 1 1
  spline S174 degree 2 poles (49.6551, 17.1287) (49.7827, 16.939) (49.8792, 16.8735) knots 0 0 0 1 1 1
  spline S175 degree 2 poles (49.8792, 16.8735) (50.0896, 16.7356) (50.4896, 16.7356) knots 0 0 0 1 1 1
  spline S176 degree 2 poles (50.4896, 16.7356) (50.8758, 16.7356) (51.2034, 16.9011) knots 0 0 0 1 1 1
  spline S177 degree 2 poles (51.2034, 16.9011) (51.6241, 17.1149) (51.6241, 17.4907) knots 0 0 0 1 1 1
  spline S178 degree 2 poles (51.6241, 17.4907) (51.6241, 17.8045) (51.2689, 17.9838) knots 0 0 0 1 1 1
  spline S179 degree 2 poles (51.2689, 17.9838) (50.9723, 18.139) (50.531, 18.1528) knots 0 0 0 1 1 1
  spline S180 degree 2 poles (50.531, 18.1528) (50.1413, 18.1666) (49.8654, 18.3252) knots 0 0 0 1 1 1
  spline S181 degree 2 poles (49.8654, 18.3252) (49.5137, 18.5252) (49.5137, 18.8976) knots 0 0 0 1 1 1
  spline S182 degree 2 poles (49.5137, 18.8976) (49.5137, 19.339) (50.0137, 19.7011) knots 0 0 0 1 1 1
  spline S183 degree 2 poles (50.0137, 19.7011) (50.4896, 20.0459) (50.9999, 20.0459) knots 0 0 0 1 1 1
  spline S184 degree 2 poles (50.9999, 20.0459) (51.2378, 20.0459) (51.5413, 19.9632) knots 0 0 0 1 1 1
  spline S185 degree 2 poles (51.5413, 19.9632) (51.9413, 19.8563) (51.9413, 19.6907) knots 0 0 0 1 1 1
  spline S186 degree 2 poles (51.9413, 19.6907) (51.9413, 19.4735) (51.7206, 19.4735) knots 0 0 0 1 1 1
  spline S187 degree 2 poles (51.7206, 19.4735) (51.6206, 19.4735) (51.1275, 19.5804) (50.9896, 19.577) knots 0 0 0 1 2 2 2
  spline S188 degree 2 poles (50.9896, 19.577) (50.6034, 19.5735) (50.3344, 19.3873) knots 0 0 0 1 1 1
  spline S189 degree 2 poles (50.3344, 19.3873) (50.0585, 19.1976) (50.0585, 18.9252) knots 0 0 0 1 1 1
  spline S190 degree 2 poles (50.0585, 18.9252) (50.0585, 18.7218) (50.4241, 18.6356) knots 0 0 0 1 1 1
  spline S191 degree 2 poles (50.4241, 18.6356) (50.562, 18.6045) (50.9516, 18.577) knots 0 0 0 1 1 1
  spline S192 degree 2 poles (50.9516, 18.577) (51.5172, 18.5356) (51.8344, 18.2218) knots 0 0 0 1 1 1
  spline S193 degree 2 poles (51.8344, 18.2218) (52.1275, 17.9356) (52.1275, 17.5218) knots 0 0 0 1 1 1
  spline S194 degree 2 poles (52.1275, 17.5218) (52.1275, 16.9321) (51.5827, 16.5804) knots 0 0 0 1 1 1
  spline S195 degree 2 poles (51.5827, 16.5804) (51.1103, 16.277) (50.4896, 16.277) knots 0 0 0 1 1 1
  spline S196 degree 2 poles (50.4896, 16.277) (50.0344, 16.277) (49.662, 16.4494) knots 0 0 0 1 1 1
  spline S197 degree 2 poles (49.662, 16.4494) (49.1999, 16.6632) (49.193, 17.0321) knots 0 0 0 1 1 1
  spline S198 degree 2 poles (52.7068, 17.0321) (52.7034, 17.1356) (52.8516, 17.2666) (52.9551, 17.2666) knots 0 0 0 1 2 2 2
  spline S199 degree 2 poles (52.9551, 17.2666) (53.0758, 17.2666) (53.1689, 17.1287) knots 0 0 0 1 1 1
  spline S200 degree 2 poles (53.1689, 17.1287) (53.2965, 16.939) (53.393, 16.8735) knots 0 0 0 1 1 1
  spline S201 degree 2 poles (53.393, 16.8735) (53.6034, 16.7356) (54.0034, 16.7356) knots 0 0 0 1 1 1
  spline S202 degree 2 poles (54.0034, 16.7356) (54.3896, 16.7356) (54.7172, 16.9011) knots 0 0 0 1 1 1
  spline S203 degree 2 poles (54.7172, 16.9011) (55.1378, 17.1149) (55.1378, 17.4907) knots 0 0 0 1 1 1
  spline S204 degree 2 poles (55.1378, 17.4907) (55.1378, 17.8045) (54.7827, 17.9838) knots 0 0 0 1 1 1
  spline S205 degree 2 poles (54.7827, 17.9838) (54.4861, 18.139) (54.0447, 18.1528) knots 0 0 0 1 1 1
  spline S206 degree 2 poles (54.0447, 18.1528) (53.6551, 18.1666) (53.3792, 18.3252) knots 0 0 0 1 1 1
  spline S207 degree 2 poles (53.3792, 18.3252) (53.0275, 18.5252) (53.0275, 18.8976) knots 0 0 0 1 1 1
  spline S208 degree 2 poles (53.0275, 18.8976) (53.0275, 19.339) (53.5275, 19.7011) knots 0 0 0 1 1 1
  spline S209 degree 2 poles (53.5275, 19.7011) (54.0034, 20.0459) (54.5137, 20.0459) knots 0 0 0 1 1 1
  spline S210 degree 2 poles (54.5137, 20.0459) (54.7516, 20.0459) (55.0551, 19.9632) knots 0 0 0 1 1 1
  spline S211 degree 2 poles (55.0551, 19.9632) (55.4551, 19.8563) (55.4551, 19.6907) knots 0 0 0 1 1 1
  spline S212 degree 2 poles (55.4551, 19.6907) (55.4551, 19.4735) (55.2344, 19.4735) knots 0 0 0 1 1 1
  spline S213 degree 2 poles (55.2344, 19.4735) (55.1344, 19.4735) (54.6413, 19.5804) (54.5034, 19.577) knots 0 0 0 1 2 2 2
  spline S214 degree 2 poles (54.5034, 19.577) (54.1172, 19.5735) (53.8482, 19.3873) knots 0 0 0 1 1 1
  spline S215 degree 2 poles (53.8482, 19.3873) (53.5723, 19.1976) (53.5723, 18.9252) knots 0 0 0 1 1 1
  spline S216 degree 2 poles (53.5723, 18.9252) (53.5723, 18.7218) (53.9378, 18.6356) knots 0 0 0 1 1 1
  spline S217 degree 2 poles (53.9378, 18.6356) (54.0758, 18.6045) (54.4654, 18.577) knots 0 0 0 1 1 1
  spline S218 degree 2 poles (54.4654, 18.577) (55.031, 18.5356) (55.3482, 18.2218) knots 0 0 0 1 1 1
  spline S219 degree 2 poles (55.3482, 18.2218) (55.6413, 17.9356) (55.6413, 17.5218) knots 0 0 0 1 1 1
  spline S220 degree 2 poles (55.6413, 17.5218) (55.6413, 16.9321) (55.0965, 16.5804) knots 0 0 0 1 1 1
  spline S221 degree 2 poles (55.0965, 16.5804) (54.6241, 16.277) (54.0034, 16.277) knots 0 0 0 1 1 1
  spline S222 degree 2 poles (54.0034, 16.277) (53.5482, 16.277) (53.1758, 16.4494) knots 0 0 0 1 1 1
  spline S223 degree 2 poles (53.1758, 16.4494) (52.7137, 16.6632) (52.7068, 17.0321) knots 0 0 0 1 1 1
  spline S224 degree 2 poles (32.4482, 8.0541) (32.4413, 7.8265) (32.2241, 7.8265) knots 0 0 0 1 1 1
  spline S225 degree 2 poles (32.2241, 7.8265) (32.0413, 7.8265) (31.962, 8.0403) knots 0 0 0 1 1 1
  line L36 (31.962, 8.0403) -> (31.5827, 9.0437)
  line L37 (31.5827, 9.0437) -> (31.1413, 10.1782)
  spline S226 degree 2 poles (31.1413, 10.1782) (31.1172, 10.2437) (31.1172, 10.292) knots 0 0 0 1 1 1
  spline S227 degree 2 poles (31.1172, 10.292) (31.1172, 10.3955) (31.2723, 10.5368) (31.3723, 10.5368) knots 0 0 0 1 2 2 2
  spline S228 degree 2 poles (31.3723, 10.5368) (31.5206, 10.5368) (31.5861, 10.3886) knots 0 0 0 1 1 1
  line L38 (31.5861, 10.3886) -> (32.2137, 8.6575)
  spline S229 degree 2 poles (32.2137, 8.6575) (32.3999, 9.0541) (32.6792, 9.8058) knots 0 0 0 1 1 1
  spline S230 degree 2 poles (32.6792, 9.8058) (32.7482, 10.0024) (32.8896, 10.3644) knots 0 0 0 1 1 1
  spline S231 degree 2 poles (32.8896, 10.3644) (32.9654, 10.523) (33.1068, 10.523) knots 0 0 0 1 1 1
  spline S232 degree 2 poles (33.1068, 10.523) (33.2103, 10.523) (33.362, 10.3782) (33.362, 10.2817) knots 0 0 0 1 2 2 2
  spline S233 degree 2 poles (33.362, 10.2817) (33.362, 10.1851) (32.9551, 9.223) knots 0 0 0 1 1 1
  line L39 (32.9551, 9.223) -> (32.4482, 8.0541)
  line L40 (35.1689, 7.923) -> (34.6792, 7.923)
  line L41 (34.6792, 7.923) -> (34.1896, 7.9265)
  spline S234 degree 2 poles (34.1896, 7.9265) (34.0172, 7.9265) (33.9482, 7.9472) knots 0 0 0 1 1 1
  spline S235 degree 2 poles (33.9482, 7.9472) (33.8206, 7.992) (33.8206, 8.1368) knots 0 0 0 1 1 1
  spline S236 degree 2 poles (33.8206, 8.1368) (33.8206, 8.3851) (34.2068, 8.3851) knots 0 0 0 1 1 1
  line L42 (34.2068, 8.3851) -> (34.3275, 8.3817)
  line L43 (34.3275, 8.3817) -> (34.4275, 8.3782)
  spline S237 degree 2 poles (34.4275, 8.3782) (34.4275, 8.4955) (34.3861, 8.961) (34.3861, 9.0782) knots 0 0 0 1 2 2 2
  spline S238 degree 2 poles (34.3861, 9.0782) (34.3861, 9.392) (34.4413, 10.0334) knots 0 0 0 1 1 1
  spline S239 degree 2 poles (34.4413, 10.0334) (34.4965, 10.661) (34.493, 10.9886) knots 0 0 0 1 1 1
  spline S240 degree 2 poles (34.493, 10.9886) (34.162, 10.7299) (34.0723, 10.7299) knots 0 0 0 1 1 1
  spline S241 degree 2 poles (34.0723, 10.7299) (33.9723, 10.7299) (33.8275, 10.8782) (33.8275, 10.9748) knots 0 0 0 1 2 2 2
  spline S242 degree 2 poles (33.8275, 10.9748) (33.8275, 11.092) (34.0413, 11.2575) knots 0 0 0 1 1 1
  spline S243 degree 2 poles (34.0413, 11.2575) (34.1723, 11.3541) (34.4172, 11.561) knots 0 0 0 1 1 1
  spline S244 degree 2 poles (34.4172, 11.561) (34.6378, 11.7817) (34.8344, 11.7817) knots 0 0 0 1 1 1
  spline S245 degree 2 poles (34.8344, 11.7817) (34.9999, 11.7817) (34.9999, 11.592) knots 0 0 0 1 1 1
  spline S246 degree 2 poles (34.9999, 11.592) (34.9999, 11.5334) (34.9689, 11.3093) (34.9689, 11.2506) knots 0 0 0 1 2 2 2
  spline S247 degree 2 poles (34.9689, 11.2506) (34.9689, 11.1713) (34.9861, 10.8403) (34.9861, 10.7575) knots 0 0 0 1 2 2 2
  spline S248 degree 2 poles (34.9861, 10.7575) (34.9861, 10.4748) (34.8689, 9.3575) (34.8689, 9.0782) knots 0 0 0 1 2 2 2
  spline S249 degree 2 poles (34.8689, 9.0782) (34.8689, 8.9334) (34.9068, 8.523) (34.9103, 8.392) knots 0 0 0 1 2 2 2
  line L44 (34.9103, 8.392) -> (35.1689, 8.3955)
  spline S250 degree 2 poles (35.1689, 8.3955) (35.2758, 8.3955) (35.4103, 8.261) (35.4103, 8.161) knots 0 0 0 1 2 2 2
  spline S251 degree 2 poles (35.4103, 8.161) (35.4103, 8.0575) (35.2758, 7.923) (35.1689, 7.923) knots 0 0 0 1 2 2 2
  spline S252 degree 2 poles (36.3689, 7.6955) (36.2413, 7.6955) (36.062, 7.8748) (36.062, 8.0024) knots 0 0 0 1 2 2 2
  spline S253 degree 2 poles (36.062, 8.0024) (36.062, 8.1299) (36.2413, 8.3093) (36.3689, 8.3093) knots 0 0 0 1 2 2 2
  spline S254 degree 2 poles (36.3689, 8.3093) (36.4965, 8.3093) (36.6758, 8.1299) (36.6758, 8.0024) knots 0 0 0 1 2 2 2
  spline S255 degree 2 poles (36.6758, 8.0024) (36.6758, 7.8748) (36.4965, 7.6955) (36.3689, 7.6955) knots 0 0 0 1 2 2 2
  spline S256 degree 2 poles (38.4827, 7.8299) (37.731, 7.8299) (37.3861, 8.5162) knots 0 0 0 1 1 1
  spline S257 degree 2 poles (37.3861, 8.5162) (37.1241, 9.0472) (37.1241, 9.8955) knots 0 0 0 1 1 1
  spline S258 degree 2 poles (37.1241, 9.8955) (37.1241, 10.6127) (37.4654, 11.1472) knots 0 0 0 1 1 1
  spline S259 degree 2 poles (37.4654, 11.1472) (37.8689, 11.7713) (38.5585, 11.7713) knots 0 0 0 1 1 1
  spline S260 degree 2 poles (38.5585, 11.7713) (39.2103, 11.7713) (39.5723, 11.2162) knots 0 0 0 1 1 1
  spline S261 degree 2 poles (39.5723, 11.2162) (39.8861, 10.7368) (39.8861, 10.0472) knots 0 0 0 1 1 1
  spline S262 degree 2 poles (39.8861, 10.0472) (39.8861, 8.9403) (39.1861, 7.8299) (38.4827, 7.8299) knots 0 0 0 1 2 2 2
  spline S263 degree 2 poles (38.5585, 11.2955) (38.0965, 11.2955) (37.8275, 10.8265) knots 0 0 0 1 1 1
  spline S264 degree 2 poles (37.8275, 10.8265) (37.6034, 10.4368) (37.6034, 9.9368) knots 0 0 0 1 1 1
  spline S265 degree 2 poles (37.6034, 9.9368) (37.6034, 9.123) (38.0447, 8.3058) (38.4827, 8.3058) knots 0 0 0 1 2 2 2
  spline S266 degree 2 poles (38.4827, 8.3058) (39.0068, 8.3058) (39.2344, 8.9058) knots 0 0 0 1 1 1
  spline S267 degree 2 poles (39.2344, 8.9058) (39.393, 9.3196) (39.393, 9.9575) knots 0 0 0 1 1 1
  spline S268 degree 2 poles (39.393, 9.9575) (39.393, 10.6265) (38.9758, 11.2955) (38.5585, 11.2955) knots 0 0 0 1 2 2 2
  spline S269 degree 2 poles (40.7241, 7.6955) (40.5965, 7.6955) (40.4172, 7.8748) (40.4172, 8.0024) knots 0 0 0 1 2 2 2
  spline S270 degree 2 poles (40.4172, 8.0024) (40.4172, 8.1299) (40.5965, 8.3093) (40.7241, 8.3093) knots 0 0 0 1 2 2 2
  spline S271 degree 2 poles (40.7241, 8.3093) (40.8516, 8.3093) (41.031, 8.1299) (41.031, 8.0024) knots 0 0 0 1 2 2 2
  spline S272 degree 2 poles (41.031, 8.0024) (41.031, 7.8748) (40.8516, 7.6955) (40.7241, 7.6955) knots 0 0 0 1 2 2 2
  spline S273 degree 2 poles (42.8378, 7.8299) (42.0861, 7.8299) (41.7413, 8.5162) knots 0 0 0 1 1 1
  spline S274 degree 2 poles (41.7413, 8.5162) (41.4792, 9.0472) (41.4792, 9.8955) knots 0 0 0 1 1 1
  spline S275 degree 2 poles (41.4792, 9.8955) (41.4792, 10.6127) (41.8206, 11.1472) knots 0 0 0 1 1 1
  spline S276 degree 2 poles (41.8206, 11.1472) (42.2241, 11.7713) (42.9137, 11.7713) knots 0 0 0 1 1 1
  spline S277 degree 2 poles (42.9137, 11.7713) (43.5654, 11.7713) (43.9275, 11.2162) knots 0 0 0 1 1 1
  spline S278 degree 2 poles (43.9275, 11.2162) (44.2413, 10.7368) (44.2413, 10.0472) knots 0 0 0 1 1 1
  spline S279 degree 2 poles (44.2413, 10.0472) (44.2413, 8.9403) (43.5413, 7.8299) (42.8378, 7.8299) knots 0 0 0 1 2 2 2
  spline S280 degree 2 poles (42.9137, 11.2955) (42.4516, 11.2955) (42.1827, 10.8265) knots 0 0 0 1 1 1
  spline S281 degree 2 poles (42.1827, 10.8265) (41.9585, 10.4368) (41.9585, 9.9368) knots 0 0 0 1 1 1
  spline S282 degree 2 poles (41.9585, 9.9368) (41.9585, 9.123) (42.3999, 8.3058) (42.8378, 8.3058) knots 0 0 0 1 2 2 2
  spline S283 degree 2 poles (42.8378, 8.3058) (43.362, 8.3058) (43.5896, 8.9058) knots 0 0 0 1 1 1
  spline S284 degree 2 poles (43.5896, 8.9058) (43.7482, 9.3196) (43.7482, 9.9575) knots 0 0 0 1 1 1
  spline S285 degree 2 poles (43.7482, 9.9575) (43.7482, 10.6265) (43.331, 11.2955) (42.9137, 11.2955) knots 0 0 0 1 2 2 2
  spline S286 degree 2 poles (45.0792, 7.6955) (44.9516, 7.6955) (44.7723, 7.8748) (44.7723, 8.0024) knots 0 0 0 1 2 2 2
  spline S287 degree 2 poles (44.7723, 8.0024) (44.7723, 8.1299) (44.9516, 8.3093) (45.0792, 8.3093) knots 0 0 0 1 2 2 2
  spline S288 degree 2 poles (45.0792, 8.3093) (45.2068, 8.3093) (45.3861, 8.1299) (45.3861, 8.0024) knots 0 0 0 1 2 2 2
  spline S289 degree 2 poles (45.3861, 8.0024) (45.3861, 7.8748) (45.2068, 7.6955) (45.0792, 7.6955) knots 0 0 0 1 2 2 2
  point P0 (38.3223, 22)
  point P1 (38.3223, 6)
  point P2 (18.3223, 15)
  point P3 (58.3223, 15)
  dimension "d0" = 112
  dimension "d1" = 112
  dimension "d2" = 135
  dimension "d3" = 135
  dimension "d4" = 135
  dimension "d8" = 25
  dimension "d313" = 40
  dimension "d314" = 16
  dimension "d315" = 6
  constraints: 6 point on line, 5 midpoint, 4 end point, 2 other
  measures "d313" distance of L0.start L0.end
  measures "d314" distance of L0.end L1.end
  measures "d315" distance between parallel lines of L9 L2
extrude "Extrusion10" cut sketch "Sketch10" against normal blind 1.5
body "Solid1"
